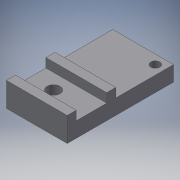
# Autodesk Inventor part: PinionHolder
Saved by Autodesk Inventor 2019 (Build 230136000, 136)
## iProperties
Created: 2019-08-06
Part Number: PinionHolder
Material: Generic
Document SubType Name: Modeling
Designer: aorfi
Density: 1 g/cm^3
Appearance: Default
Author: aorfi
Autodesk Inventor part; units mm, degrees
ref_plane "YZ Plane" through (0, 0, 0) normal (1, 0, 0) x (0, 1, 0)
ref_plane "XZ Plane" through (0, 0, 0) normal (0, 1, 0) x (-1, 0, 0)
ref_plane "XY Plane" through (0, 0, 0) normal (0, 0, 1) x (1, 0, 0)
sketch "Sketch1" plane through (0, 0, 0) normal (0, 1, 0) x (-1, 0, 0)
  line L0 (10, 17.5) -> (-10, 17.5)
  line L1 (-10, 17.5) -> (-10, -17.5)
  line L2 (-10, -17.5) -> (10, -17.5)
  line L3 (10, -17.5) -> (10, 17.5)
  line L4 (10, 17.5) -> (-10, -17.5) construction
  line L5 (-10, 17.5) -> (10, -17.5) construction
  point P0 (0, 0)
  dimension "d2" = 20
  dimension "d3" = 35
  constraints: 12 end point, 2 midpoint, 2 parallel, 1 horizontal, 1 perpendicular
  measures "d2" distance of L1.end L2.end
  measures "d3" distance of L0.end L1.end
extrude "Extrusion1" add sketch "Sketch1" along normal mid plane 5
sketch "Sketch2" plane through (0, 2.5, 0) normal (0, 1, 0) x (1, 0, 0)
  line L0 (10, -1.5) -> (-10, -1.5)
  line L1 (-10, -1.5) -> (-10, -4.5)
  line L2 (-10, -4.5) -> (10, -4.5)
  line L3 (10, -4.5) -> (10, -1.5)
  line L4 (10, -14.5) -> (-10, -14.5)
  line L5 (-10, -14.5) -> (-10, -17.5)
  line L6 (-10, -17.5) -> (10, -17.5)
  line L7 (10, -17.5) -> (10, -14.5)
  line L8 (10, -17.5) -> (10, 17.5) projected
  line L9 (-10, 17.5) -> (-10, -17.5) projected
  line L10 (10, 17.5) -> (-10, 17.5) projected
  line L11 (-10, -17.5) -> (10, -17.5) projected
  point P0 (0, 0)
  dimension "d4" = 3
  dimension "d5" = 3
  dimension "d6" = 10
  constraints: 16 end point, 5 collinear, 4 parallel, 2 horizontal, 2 perpendicular
  measures "d4" distance of L2.end L0.start
  measures "d5" distance of L6.end L4.start
  measures "d6" distance between parallel lines of L4 L2
extrude "Extrusion2" add sketch "Sketch2" along normal blind 3 contours L3 L2 L1 L0 | L7 L6 L5 L4
sketch "Sketch3" plane through (0, 2.5, 0) normal (0, 1, 0) x (1, 0, 0)
  line L0 (10, -4.5) -> (-10, -4.5) projected
  line L1 (-10, -4.5) -> (-10, -14.5) projected
  line L2 (-10, -14.5) -> (10, -14.5) projected
  line L3 (10, -14.5) -> (10, -4.5) projected
  line L4 (10, -14.5) -> (-10, -14.5) projected
  point P0 (0, 0)
  point P1 (-2.5, -9.5)
  point P2 (-10, -9.5)
  point P3 (0, -14.5)
  dimension "d26" = 12.5
  constraints: 2 midpoint, 1 horizontal alignment
  measures "d26" distance from line of L3 point (-2.5, -9.5)
hole "Hole1" at (-2.5, 2.5, 9.5) direction (0, -1, 0) diameter 4.305 end through all clearance for "Flat Head Machine Screw (82)" size "#6" standard "Ansi Unified Screw Threads"
sketch "Sketch4" plane through (0, -2.5, 0) normal (0, -1, 0) x (1, 0, 0)
  circle A0 centre (-2.5, -6.977) radius 3.9688
  circle A1 centre (-2.5, 9.5) radius 2.1525 projected
  point P0 (0, 0)
  dimension "d16" = 7.9375
  dimension "d17" = 16.477
  constraints: 1 centre point, 1 vertical alignment
  measures "d16" diameter of A0
  measures "d17" distance of A0.centre A1.centre
extrude "Extrusion3" add sketch "Sketch4" along normal blind 5 contours A0
sketch "Sketch5" plane through (0, -2.5, 0) normal (0, -1, 0) x (1, 0, 0)
  circle A0 centre (7, -14.5) radius 1.5
  line L0 (-10, -17.5) -> (10, -17.5) projected
  line L1 (-10, 17.5) -> (-10, -17.5) projected
  line L2 (10, -17.5) -> (10, 17.5) projected
  point P0 (0, 0)
  dimension "d20" = 3
  dimension "d21" = 3
  dimension "d25" = 3
  constraints: 1 centre point
  measures "d20" diameter of A0
  measures "d21" distance from line of L0 A0.centre
  measures "d25" distance from line of L2 A0.centre
extrude "Extrusion4" cut sketch "Sketch5" against normal through all
equation "\"d5\" = d4"
body "Solid1"
